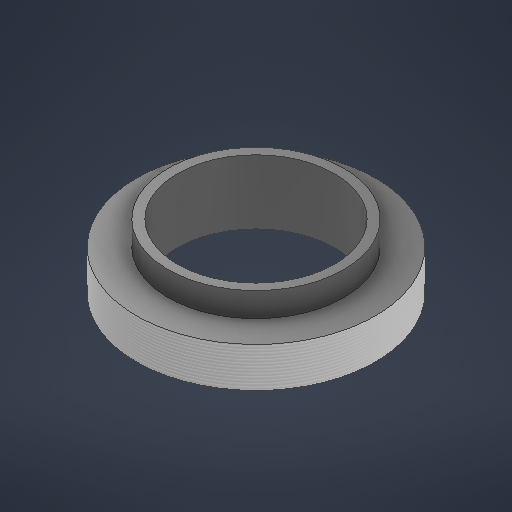
# Autodesk Inventor part: 38mm to SM2
Saved by Autodesk Inventor 2026 (Build 300175000, 175)
## iProperties
Created: 2025-11-11
Part Number: 38mm to SM2
Material: Aluminum 6061-AHC
Document SubType Name: Modeling
Designer: FiolkaLab
Density: 2.7 g/cm^3
Appearance: Aluminum - Dark
Mass: 16.867 g
Surface Area: 47.1256 cm^2
Volume: 6.24703 cm^3
Author: FiolkaLab
Autodesk Inventor part; units mm, degrees
ref_plane "YZ Plane" through (0, 0, 0) normal (1, 0, 0) x (0, 1, 0)
ref_plane "XZ Plane" through (0, 0, 0) normal (0, 1, 0) x (-1, 0, 0)
ref_plane "XY Plane" through (0, 0, 0) normal (0, 0, 1) x (1, 0, 0)
sketch "Sketch1" plane through (0, 0, 0) normal (0, 1, 0) x (-1, 0, 0)
  circle A0 centre (0, 0) radius 25.8445
  dimension "d0" = 51.689
  constraints: 1 centre point, 1 coincident
  measures "d0" diameter of A0
extrude "Extrusion1" add sketch "Sketch1" along normal blind 8.636
sketch "Sketch2" plane through (0, 8.636, 0) normal (0, 1, 0) x (1, 0, 0)
  circle A0 centre (0, 0) radius 19
  dimension "d3" = 37.9999
  constraints: 1 centre point, 1 coincident
  measures "d3" diameter of A0
extrude "Extrusion2" add sketch "Sketch2" along normal blind 5.25
sketch "Sketch3" plane through (0, 13.886, 0) normal (0, 1, 0) x (1, 0, 0)
  circle A0 centre (0, 0) radius 17
  dimension "d6" = 33.9999
  constraints: 1 centre point, 1 coincident
  measures "d6" diameter of A0
extrude "Extrusion3" cut sketch "Sketch3" against normal through all
thread "Thread2" size "2.035-40 UNS" designation "SM2 (2.035-40 UNS)" class "2A" standard "ANSI Unified Screw Threads" full length
body "Solid1"
